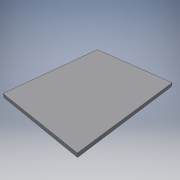
# Autodesk Inventor part: support platforms (for assembly)
Saved by Autodesk Inventor 2016 (Build 200138000, 138)
## iProperties
Created: 2017-10-23
Part Number: support platforms (for assembly)
Material: Generic
Document SubType Name: Modeling
Designer: student
Density: 1 g/cm^3
Appearance: Default
Author: student
Autodesk Inventor part; units mm, degrees
ref_plane "YZ Plane" through (0, 0, 0) normal (1, 0, 0) x (0, 1, 0)
ref_plane "XZ Plane" through (0, 0, 0) normal (0, 1, 0) x (-1, 0, 0)
ref_plane "XY Plane" through (0, 0, 0) normal (0, 0, 1) x (1, 0, 0)
sketch "Sketch1" plane through (0, 0, 0) normal (0, 1, 0) x (-1, 0, 0)
  line L0 (-203.2, 254) -> (203.2, 254)
  line L1 (203.2, 254) -> (203.2, -254)
  line L2 (203.2, -254) -> (-203.2, -254)
  line L3 (-203.2, -254) -> (-203.2, 254)
  line L4 (-203.2, 254) -> (203.2, -254) construction
  line L5 (203.2, 254) -> (-203.2, -254) construction
  point P0 (0, 0)
  dimension "d0" = 406.4
  dimension "d1" = 508
  constraints: 12 end point, 2 midpoint, 2 parallel, 1 horizontal, 1 perpendicular
  measures "d0" distance of L1.end L2.end
  measures "d1" distance of L0.end L1.end
extrude "Extrusion1" add sketch "Sketch1" along normal blind 19.05
body "Solid1"
